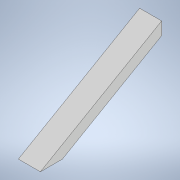
# Autodesk Inventor part: КРЫШАДЕТАЛЬXI
Saved by Autodesk Inventor 2022.4 (Build 264492010, 492A)
## iProperties
Created: 2023-02-19
Part Number: КРЫШАДЕТАЛЬXI
Material: Типовые
Document SubType Name: Modeling
Designer: artyo
Density: 1 g/cm^3
Appearance: По умолчанию
Author: artyo
Autodesk Inventor part; units mm, degrees
ref_plane "YZ Plane" through (0, 0, 0) normal (1, 0, 0) x (0, 1, 0)
ref_plane "XZ Plane" through (0, 0, 0) normal (0, 1, 0) x (-1, 0, 0)
ref_plane "XY Plane" through (0, 0, 0) normal (0, 0, 1) x (1, 0, 0)
sketch "Эскиз4" plane through (0, 0, 0) normal (0, 1, 0) x (-1, 0, 0)
  line L0 (-10, -10) -> (10, -10)
  line L1 (10, -10) -> (10, 10)
  line L2 (10, 10) -> (-10, 10)
  line L3 (-10, 10) -> (-10, -10)
  line L4 (-10, -10) -> (10, 10) construction
  line L5 (10, -10) -> (-10, 10) construction
  line L6 (-9.25, -9.25) -> (9.25, -9.25)
  line L7 (9.25, -9.25) -> (9.25, 9.25)
  line L8 (9.25, 9.25) -> (-9.25, 9.25)
  line L9 (-9.25, 9.25) -> (-9.25, -9.25)
  line L10 (-9.25, -9.25) -> (9.25, 9.25) construction
  line L11 (9.25, -9.25) -> (-9.25, 9.25) construction
  point P0 (0, 0)
  dimension "d11" = 20
  dimension "d12" = 20
  dimension "d13" = 18.5
  dimension "d14" = 18.5
  constraints: 24 end point, 4 midpoint, 4 parallel, 2 horizontal, 2 perpendicular
  measures "d11" distance of L2.end L1.end
  measures "d12" distance of L1.end L0.end
  measures "d13" distance of L8.end L7.end
  measures "d14" distance of L7.end L6.end
sketch "Эскиз5" plane through (0, 0, 0) normal (1, 0, 0) x (0, 1, 0)
  line L0 (0, 0) -> (63.5, -109.9852)
  line L1 (0, 0) -> (127, 0) construction
  dimension "d15" = 127
  dimension "d16" = 60
  constraints: 4 end point, 1 equal length, 1 horizontal
  measures "d15" distance of L0.start L0.end
  measures "d16" angle of L0 L1
sweep "Сдвиг1" add profiles "Эскиз4" path "Эскиз5"
sketch "Эскиз6" plane through (10, 0, 10) normal (1, 0, 0) x (0, 0, -1)
  line L0 (109.9852, 63.5) -> (119.9852, 57.7265)
  line L1 (20, 0) -> (129.9852, 63.5) projected
  line L2 (109.9852, 63.5) -> (121.5322, 63.5) construction
  line L3 (119.9852, 57.7265) -> (129.9852, 63.5)
  line L4 (129.9852, 63.5) -> (109.9852, 63.5)
  line L5 (129.2352, 63.5) -> (110.7352, 63.5) projected
  point P0 (10, 0)
  dimension "d19" = 30
  constraints: 8 end point, 2 collinear, 1 equal length, 1 horizontal, 1 point on line
  measures "d19" angle of L0 L2
extrude "Выдавливание3" cut sketch "Эскиз6" against normal blind 127.0171
sketch "Эскиз7" plane through (10, 0, 10) normal (1, 0, 0) x (0, 0, -1)
  line L0 (0, 0) -> (109.9852, 63.5) projected
  line L1 (109.9852, 63.5) -> (109.9852, 51.953)
  line L2 (20, 0) -> (119.9852, 57.7265) projected
  line L3 (109.9852, 63.5) -> (119.9852, 57.7265)
  line L4 (109.9852, 51.953) -> (109.9852, 51.4136)
  line L5 (109.9852, 51.4136) -> (120.7731, 57.642)
  line L6 (20, 0) -> (119.9852, 57.7265) projected
  line L7 (119.9852, 57.7265) -> (120.7731, 57.2716)
  point P0 (10, 0)
  point P1 (120.4523, 57.4568)
  constraints: 10 end point, 2 vertical, 1 parallel, 1 point on line
extrude "Выдавливание4" cut sketch "Эскиз7" against normal blind 127.0171
